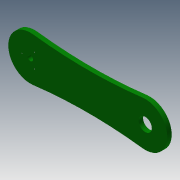
# Autodesk Inventor part: rameno(a)nahore
Saved by Autodesk Inventor 2013 (Build 170138000, 138)
## iProperties
Created: 2013-05-25
Part Number: rameno(a)nahore
Material: Generic
Document SubType Name: Modeling
Designer: idle-rug
Density: 1 g/cm^3
Author: idle-rug
Autodesk Inventor part; units mm, degrees
ref_plane "YZ Plane" through (0, 0, 0) normal (1, 0, 0) x (0, 1, 0)
ref_plane "XZ Plane" through (0, 0, 0) normal (0, 1, 0) x (-1, 0, 0)
ref_plane "XY Plane" through (0, 0, 0) normal (0, 0, 1) x (1, 0, 0)
sketch "Sketch1" plane through (0, 0, 0) normal (0, 1, 0) x (-1, 0, 0)
  line L0 (-75, -25) -> (75, -25)
  line L1 (75, -25) -> (75, 25)
  line L2 (75, 25) -> (-75, 25)
  line L3 (-75, 25) -> (-75, -25)
  line L4 (-75, -25) -> (75, 25) construction
  line L5 (75, -25) -> (-75, 25) construction
  circle A0 centre (75, 0) radius 25
  circle A1 centre (-75, 0) radius 25
  point P0 (0, 0)
  dimension "d0" = 150
  dimension "d1" = 50
  constraints: 12 end point, 4 midpoint, 2 parallel, 2 vertical alignment, 1 horizontal, 1 perpendicular, 4 other
  measures "d0" distance of L2.end L1.end
  measures "d1" distance of L1.end L0.end
extrude "Extrusion1" add sketch "Sketch1" along normal blind 5
sketch "Sketch2" plane through (0, 5, 0) normal (0, 1, 0) x (1, 0, 0)
  arc A0 (75, -25) -> (75, 25) centre (75, 0) ccw projected
  arc A1 (-75, 25) -> (-75, -25) centre (-75, 0) ccw projected
  circle A2 centre (-75, 0) radius 3
  circle A3 centre (75, 0) radius 3
  point P0 (0, 0)
  dimension "d4" = 6
  dimension "d5" = 6
  constraints: 2 centre point, 2 coincident
  measures "d4" diameter of A2
  measures "d5" diameter of A3
extrude "Extrusion2" cut sketch "Sketch2" against normal blind 5
sketch "Sketch3" plane through (0, 5, 0) normal (0, 1, 0) x (1, 0, 0)
  line L0 (75, 25) -> (-75, 25) projected
  line L1 (-41.092, 0) -> (-59.192, 0)
  line L2 (-59.192, 0) -> (-4.192, 0)
  line L3 (-4.192, 10) -> (-59.192, 10)
  line L4 (-59.192, 10) -> (-59.192, -10)
  line L5 (-59.192, -10) -> (-4.192, -10)
  line L6 (-4.192, -10) -> (-4.192, 10)
  line L7 (-11.592, 10) -> (-51.792, 10)
  line L8 (-51.792, 10) -> (-51.792, -10)
  line L9 (-51.792, -10) -> (-11.592, -10)
  line L10 (-11.592, -10) -> (-11.592, 10)
  circle A0 centre (-6.842, 4.95) radius 1.5
  circle A1 centre (-6.842, -4.95) radius 1.5
  circle A2 centre (-56.542, 4.95) radius 1.5
  circle A3 centre (-56.542, -4.95) radius 1.5
  point P0 (0, 0)
  point P1 (-31.692, 0)
  point P2 (-51.792, 0)
  point P3 (-11.592, 0)
  dimension "d11" = 55
  dimension "d12" = 20
  dimension "d13" = 40.2
  dimension "d14" = 20
  dimension "d20" = 3
  dimension "d21" = 3
  dimension "d22" = 3
  constraints: 20 end point, 5 parallel, 4 centre point, 3 midpoint, 2 horizontal, 2 perpendicular, 1 collinear
  measures "d11" distance of L5.end L4.end
  measures "d12" distance of L4.end L3.end
  measures "d13" distance of L9.end L8.end
  measures "d14" distance of L8.end L7.end
  measures "d20" diameter of A1
  measures "d21" diameter of A2
  measures "d22" diameter of A3
extrude "Extrusion3" cut sketch "Sketch3" against normal blind 5 contours L2 L10 L5 L8 L1 | L1 L8 L3 L10 L2
sketch "Sketch4" plane through (0, 0, 0) normal (0, -1, 0) x (1, 0, 0)
  circle A0 centre (75, 0) radius 3 projected
  line L0 (-75, 25) -> (75, 25) projected
  circle A1 centre (75, 0) radius 17.325
  line L1 (78, 0) -> (92.325, 0)
  circle A2 centre (85.1625, 0) radius 1.5
  line L2 (75, 0) -> (92.325, 0) construction
  line L3 (75, 0) -> (92.325, 0) construction
  circle A3 centre (69.9187, 8.801) radius 1.5
  circle A4 centre (69.9187, -8.801) radius 1.5
  point P0 (0, 0)
  constraints: 6 end point, 3 centre point, 2 horizontal, 2 horizontal alignment, 1 midpoint, 1 parallel, 3 other
extrude "Extrusion4" cut sketch "Sketch4" against normal blind 5 contours A2 L1 | L1 A2 | A3 | A4
sketch "Sketch5" plane through (0, 0, 0) normal (0, -1, 0) x (1, 0, 0)
  circle A0 centre (69.9187, 8.801) radius 1.5 projected
  circle A1 centre (85.1625, 0) radius 1.5 projected
  circle A2 centre (69.9187, -8.801) radius 1.5 projected
  circle A3 centre (69.9187, 8.801) radius 0.5
  circle A4 centre (85.1625, 0) radius 0.5
  circle A5 centre (69.9187, -8.801) radius 0.5
  point P0 (0, 0)
  dimension "d34" = 1
  dimension "d35" = 1
  dimension "d36" = 1
  constraints: 3 centre point, 3 coincident
  measures "d34" diameter of A3
  measures "d35" diameter of A4
  measures "d36" diameter of A5
extrude "Extrusion5" add sketch "Sketch5" against normal blind 5
sketch "Sketch6" plane through (0, 0, 0) normal (0, -1, 0) x (1, 0, 0)
  circle A0 centre (-75, 0) radius 3 projected
  circle A1 centre (75, 0) radius 3 projected
  arc A2 (75, -25) -> (75, 25) centre (75, 0) ccw projected
  arc A3 (-75, 25) -> (-75, -25) centre (-75, 0) ccw projected
  circle A4 centre (75, 0) radius 7.5
  circle A5 centre (-75, 0) radius 7.5
  point P0 (0, 0)
  dimension "d39" = 15
  dimension "d40" = 15
  constraints: 2 centre point, 2 coincident
  measures "d39" diameter of A4
  measures "d40" diameter of A5
extrude "Extrusion6" cut sketch "Sketch6" against normal blind 5
sketch "Sketch7" plane through (0, 0, 0) normal (0, -1, 0) x (1, 0, 0)
  circle A0 centre (69.9187, -8.801) radius 0.5 projected
  circle A1 centre (69.9187, 8.801) radius 0.5 projected
  arc A2 (75, -25) -> (75, 25) centre (75, 0) ccw projected
  line L0 (75, 0) -> (69.9187, 8.801)
  line L1 (69.9187, -8.801) -> (75, 0)
  circle A3 centre (70.0438, 8.5845) radius 0.5
  circle A4 centre (84.9125, 0) radius 0.5
  circle A5 centre (70.0438, -8.5845) radius 0.5
  point P0 (0, 0)
  dimension "d44" = 1
  dimension "d45" = 1
  dimension "d46" = 1
  constraints: 4 end point, 3 centre point, 2 point on line, 1 coincident
  measures "d44" diameter of A3
  measures "d45" diameter of A4
  measures "d46" diameter of A5
sketch "Sketch8" plane through (0, 0, 0) normal (0, -1, 0) x (1, 0, 0)
  circle A0 centre (69.9187, -8.801) radius 0.5 projected
  circle A1 centre (69.9187, 8.801) radius 0.5 projected
  circle A2 centre (85.1625, 0) radius 0.5 projected
  point P0 (0, 0)
extrude "Extrusion7" add sketch "Sketch8" against normal blind 5
extrude "Extrusion8" cut sketch "Sketch7" against normal blind 5 contours A0 A5 | A0 L1 A5 | A0 A5 L1 | A1 A3 | A1 A3 L0 | L0 A3 A1 | A4 picked at (69.9199, -8.7989) picked at (69.9199, 8.7989)
sketch "Sketch9" plane through (0, 5, 0) normal (0, 1, 0) x (1, 0, 0)
  circle A0 centre (-75, 0) radius 7.5 projected
  line L0 (-51.792, -10) -> (-51.792, 10) projected
  line L1 (-51.792, 10) -> (-11.592, 10) projected
  line L2 (-11.592, 10) -> (-11.592, -10) projected
  line L3 (-11.592, -10) -> (-51.792, -10) projected
  line L4 (-11.592, 0) -> (-51.792, 0)
  point P0 (0, 0)
  constraints: 2 end point, 2 midpoint
extrude "Extrusion9" add sketch "Sketch9" against normal blind 5
sketch "Sketch10" plane through (0, 5, 0) normal (0, 1, 0) x (1, 0, 0)
  line L0 (-75, -25) -> (75, -25) projected
  arc A0 (75, -25) -> (75, 25) centre (75, 0) ccw projected
  line L1 (75, 25) -> (-75, 25) projected
  line L2 (75, 0) -> (-55, 0)
  circle A1 centre (-55, 0) radius 25
  arc A2 (-75, 25) -> (-75, -25) centre (-75, 0) ccw
  line L3 (-75, 25) -> (-55, 25)
  line L4 (-75, -25) -> (-55, -25)
  arc A3 (-55, 25) -> (-55, -25) centre (-55, 0) ccw
  point P0 (0, 0)
  dimension "d53" = 130
  constraints: 6 end point, 6 point on circle, 5 tangent, 3 centre point, 2 point on line, 1 coincident, 1 parallel
  measures "d53" distance of L2.start L2.end
extrude "Extrusion10" cut sketch "Sketch10" against normal blind 5 contours A2 L1 A1 L0
sketch "Sketch11" plane through (0, 5, 0) normal (0, 1, 0) x (1, 0, 0)
  arc A0 (-55, 25) -> (-55, -25) centre (-55, 0) ccw projected
  line L0 (75, 25) -> (-55, 25) projected
  circle A1 centre (-55, 0) radius 7.5
  line L1 (-55, 0) -> (-11.692, 0)
  line L2 (8.408, 10) -> (-31.792, 10)
  line L3 (-31.792, 10) -> (-31.792, -10)
  line L4 (-31.792, -10) -> (8.408, -10)
  line L5 (8.408, -10) -> (8.408, 10)
  line L6 (8.408, 10) -> (-31.792, -10) construction
  line L7 (-31.792, 10) -> (8.408, -10) construction
  point P0 (0, 0)
  dimension "d56" = 15
  dimension "d57" = 43.308
  dimension "d58" = 40.2
  dimension "d59" = 20
  constraints: 14 end point, 3 parallel, 2 midpoint, 1 centre point, 1 coincident, 1 horizontal, 1 perpendicular
  measures "d56" diameter of A1
  measures "d57" distance of L1.start L1.end
  measures "d58" distance of L4.end L3.end
  measures "d59" distance of L3.end L2.end
extrude "Extrusion11" cut sketch "Sketch11" against normal blind 5
sketch "Sketch12" plane through (0, 5, 0) normal (0, 1, 0) x (1, 0, 0)
  arc A0 (-55, 25) -> (-55, -25) centre (-55, 0) ccw projected
  line L0 (75, 25) -> (-55, 25) projected
  line L1 (-55, 0) -> (-21.85, 0)
  line L2 (-21.85, 0) -> (-39.95, 0)
  line L3 (-39.95, 0) -> (15.05, 0)
  line L4 (7.65, 10) -> (-32.55, 10)
  line L5 (-32.55, 10) -> (-32.55, -10)
  line L6 (-32.55, -10) -> (7.65, -10)
  line L7 (7.65, -10) -> (7.65, 10)
  line L8 (7.65, 10) -> (-32.55, -10) construction
  line L9 (-32.55, 10) -> (7.65, -10) construction
  line L10 (7.65, -10) -> (8.408, -10)
  line L11 (8.408, -10) -> (8.408, 10)
  line L12 (8.408, 10) -> (7.65, 10)
  line L13 (7.65, 10) -> (7.65, -10)
  line L14 (-32.55, -10) -> (-31.792, -10)
  line L15 (-31.792, -10) -> (-31.792, 10)
  line L16 (-31.792, 10) -> (-32.55, 10)
  line L17 (-32.55, 10) -> (-32.55, -10)
  point P0 (0, 0)
  point P1 (-12.45, 0)
  dimension "d62" = 33.15
  dimension "d63" = 18.1
  dimension "d64" = 55
  dimension "d65" = 40.2
  dimension "d66" = 20
  constraints: 34 end point, 7 parallel, 3 horizontal, 3 midpoint, 3 perpendicular, 2 point on line
  measures "d62" distance of L1.start L1.end
  measures "d63" distance of L1.end L2.end
  measures "d64" distance of L2.end L3.end
  measures "d65" distance of L6.end L5.end
  measures "d66" distance of L5.end L4.end
extrude "Extrusion12" add sketch "Sketch12" against normal blind 5 contours L5 L4 L15 L1 | L1 L15 L6 L5 | L7 L12 L11 L3 | L3 L11 L10 L7
sketch "Sketch14" plane through (0, 5, 0) normal (0, 1, 0) x (1, 0, 0)
  line L0 (7.65, -10) -> (-31.792, -10) projected
  circle A0 centre (-55, 0) radius 7.5 projected
  line L1 (-55, 0) -> (-21.85, 0)
  line L2 (-21.85, 0) -> (-39.95, 0)
  line L3 (-39.95, 0) -> (15.05, 0)
  line L4 (-32.55, -10) -> (7.65, -10)
  line L5 (7.65, -10) -> (7.65, 10)
  line L6 (7.65, 10) -> (-32.55, 10)
  line L7 (-32.55, 10) -> (-32.55, -10)
  line L8 (-32.55, -10) -> (7.65, 10) construction
  line L9 (7.65, -10) -> (-32.55, 10) construction
  line L10 (-32.55, -10) -> (-31.792, -10)
  line L11 (-31.792, -10) -> (-31.792, 10)
  line L12 (-31.792, 10) -> (-32.55, 10)
  line L13 (-32.55, 10) -> (-32.55, -10)
  point P0 (0, 0)
  point P1 (-12.45, 0)
  dimension "d69" = 33.15
  dimension "d70" = 18.1
  dimension "d71" = 55
  dimension "d72" = 40.2
  dimension "d73" = 20
  constraints: 26 end point, 5 parallel, 3 midpoint, 2 horizontal, 2 perpendicular, 2 point on line
  measures "d69" distance of L1.start L1.end
  measures "d70" distance of L1.end L2.end
  measures "d71" distance of L2.end L3.end
  measures "d72" distance of L6.end L5.end
  measures "d73" distance of L5.end L4.end
extrude "Extrusion13" cut sketch "Sketch14" against normal blind 5 contours L4 L7 L1 L11 | L1 L7 L6 L11
sketch "Sketch15" plane through (0, 5, 0) normal (0, 1, 0) x (1, 0, 0)
  line L0 (7.65, -10) -> (-32.55, -10) projected
  line L1 (-32.55, -10) -> (-32.55, 10) projected
  line L2 (-32.55, 10) -> (7.65, 10) projected
  line L3 (7.65, 10) -> (7.65, -10) projected
  point P0 (0, 0)
extrude "Extrusion14" add sketch "Sketch15" against normal blind 5
sketch "Sketch16" plane through (0, 0, 0) normal (0, -1, 0) x (1, 0, 0)
  circle A0 centre (-55, 0) radius 7.5 projected
  arc A1 (-55, 25) -> (-55, -25) centre (-55, 0) ccw projected
  arc A2 (75, -25) -> (75, 25) centre (75, 0) ccw projected
  circle A3 centre (84.9125, 0) radius 0.5 projected
  circle A4 centre (70.0438, -8.5845) radius 0.5 projected
  circle A5 centre (70.0438, 8.5845) radius 0.5 projected
  circle A6 centre (75, 0) radius 7.5 projected
  line L0 (75, 0) -> (-55, 0)
  line L1 (100, 0) -> (-80, 0)
  line L2 (-55, -25) -> (75, -25)
  line L3 (75, -25) -> (-55, -25) projected
  arc A7 (-51.9048, 24.8077) -> (71.9048, 24.8077) centre (10, 520.9607) ccw
  arc A8 (71.9048, -24.8077) -> (-51.9048, -24.8077) centre (10, -520.9607) ccw
  arc A9 (-51.9048, 24.8077) -> (-51.9048, -24.8077) centre (-55, 0) ccw
  arc A10 (71.9048, -24.8077) -> (71.9048, 24.8077) centre (75, 0) ccw
  point P0 (0, 0)
  constraints: 10 point on circle, 6 end point, 4 centre point, 4 tangent, 3 symmetric about line, 2 coincident, 1 collinear, 1 concentric, 1 other
extrude "Extrusion15" add sketch "Sketch16" along normal blind 5 contours L0 A6 L1 A3 A2 A10 A8 A9 A1 A0 | A0 L1 A1 A9 A7 A10 A2 A3 A6 L0
sketch "Sketch17" plane through (0, 5, 0) normal (0, 1, 0) x (1, 0, 0)
  circle A0 centre (-55, 0) radius 7.5 projected
  arc A1 (-55, 25) -> (-55, -25) centre (-55, 0) ccw projected
  line L0 (-55, -25) -> (75, -25) projected
  arc A2 (75, -25) -> (75, 25) centre (75, 0) ccw projected
  line L1 (75, 25) -> (-55, 25) projected
  circle A3 centre (75, 0) radius 7.5 projected
  circle A4 centre (70.0438, -8.5845) radius 0.5 projected
  circle A5 centre (70.0438, 8.5845) radius 0.5 projected
  circle A6 centre (84.9125, 0) radius 0.5 projected
  point P0 (0, 0)
extrude "Extrusion16" cut sketch "Sketch17" against normal blind 5
sketch "Sketch19" plane through (0, -5, 0) normal (0, -1, 0) x (1, 0, 0)
  circle A0 centre (-55, 0) radius 7.5 projected
  arc A1 (-51.9048, 24.8077) -> (-51.9048, -24.8077) centre (-55, 0) ccw projected
  circle A2 centre (-55, 0) radius 3
  point P0 (0, 0)
  dimension "d98" = 6
  constraints: 1 centre point, 1 coincident
  measures "d98" diameter of A2
extrude "Extrusion18" add sketch "Sketch19" against normal blind 5
sketch "Sketch20" plane through (0, -5, 0) normal (0, -1, 0) x (1, 0, 0)
  arc A0 (-51.9048, 24.8077) -> (-51.9048, -24.8077) centre (-55, 0) ccw projected
  circle A1 centre (-55, 0) radius 9.5375
  circle A2 centre (-64.5375, 0) radius 1
  line L0 (-55, 0) -> (-50.2313, 8.2597)
  line L1 (-55, 0) -> (-45.4625, 0) construction
  line L2 (-55, 0) -> (-50.2313, -8.2597)
  line L3 (-55, 0) -> (-45.4625, 0) construction
  circle A3 centre (-50.2313, 8.2597) radius 1
  circle A4 centre (-50.2313, -8.2597) radius 1
  point P0 (0, 0)
  dimension "d101" = 19.075
  dimension "d102" = 2
  dimension "d103" = 60
  dimension "d104" = 60
  dimension "d105" = 2
  dimension "d106" = 2
  constraints: 8 end point, 4 centre point, 3 coincident, 3 point on circle, 2 equal length, 2 horizontal
  measures "d101" diameter of A1
  measures "d102" diameter of A2
  measures "d103" angle of L1 L0
  measures "d104" angle of L2 L3
  measures "d105" diameter of A3
  measures "d106" diameter of A4
extrude "Extrusion19" cut sketch "Sketch20" against normal blind 5 contours A3 L0 A1 | A1 A3 | A4 A1 | A1 L2 A4 | L0 A3 A1 | A1 A4 L2 | A2 A1 | A1 A2
sketch "Sketch21" plane through (0, -5, 0) normal (0, -1, 0) x (1, 0, 0)
  circle A0 centre (-50.2313, -8.2597) radius 1 projected
  circle A1 centre (-64.5375, 0) radius 1 projected
  circle A2 centre (-50.2313, 8.2597) radius 1 projected
  circle A3 centre (-50.2313, 8.2597) radius 0.5
  circle A4 centre (-64.5375, 0) radius 0.5
  circle A5 centre (-50.2313, -8.2597) radius 0.5
  point P0 (0, 0)
  dimension "d109" = 1
  dimension "d110" = 1
  dimension "d111" = 1
  constraints: 3 centre point, 3 coincident
  measures "d109" diameter of A3
  measures "d110" diameter of A4
  measures "d111" diameter of A5
extrude "Extrusion20" add sketch "Sketch21" against normal blind 5
sketch "Sketch22" plane through (0, -5, 0) normal (0, -1, 0) x (1, 0, 0)
  circle A0 centre (70.0438, -8.5845) radius 0.5 projected
  circle A1 centre (70.0438, 8.5845) radius 0.5 projected
  circle A2 centre (84.9125, 0) radius 0.5 projected
  point P0 (0, 0)
extrude "Extrusion21" add sketch "Sketch22" against normal blind 5
body "Solid1"
